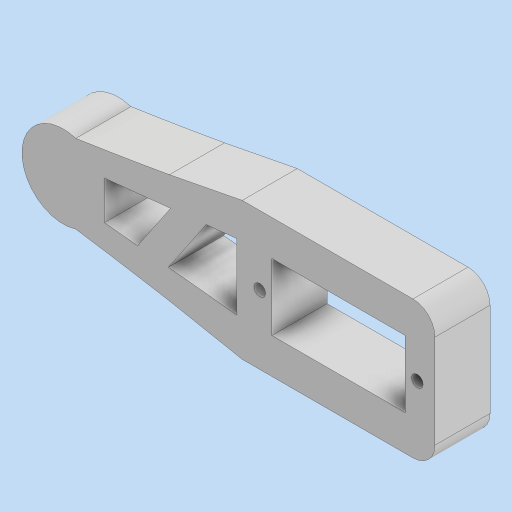
# Autodesk Inventor part: pata_inferior_v3
Saved by Autodesk Inventor 2024 (Build 280153000, 153)
## iProperties
Created: 2024-08-03
Part Number: pata_inferior_v3
Material: Generic
Document SubType Name: Modeling
Designer: MxMon
Density: 1 g/cm^3
Appearance: Default
Author: MxMon
Autodesk Inventor part; units mm, degrees
ref_plane "YZ Plane" through (0, 0, 0) normal (1, 0, 0) x (0, 1, 0)
ref_plane "XZ Plane" through (0, 0, 0) normal (0, 1, 0) x (-1, 0, 0)
ref_plane "XY Plane" through (0, 0, 0) normal (0, 0, 1) x (1, 0, 0)
sketch "Sketch1" plane through (0, 0, 0) normal (0, 0, 1) x (1, 0, 0)
  line L0 (-12.1, 6.05) -> (12.1, 6.05)
  line L1 (12.1, 6.05) -> (12.1, -6.05)
  line L2 (12.1, -6.05) -> (-12.1, -6.05)
  line L3 (-12.1, -6.05) -> (-12.1, 6.05)
  line L4 (-12.1, 6.05) -> (12.1, -6.05) construction
  line L5 (12.1, 6.05) -> (-12.1, -6.05) construction
  line L6 (-17.5, 12.5) -> (17.5, 12.5)
  line L7 (17.5, 12.5) -> (17.5, -12.5)
  line L8 (17.5, -12.5) -> (-17.5, -12.5)
  line L9 (-17.5, 12.5) -> (17.5, -12.5) construction
  line L10 (17.5, 12.5) -> (-17.5, -12.5) construction
  arc A0 (-43.9311, 7.3622) -> (-43.9311, -7.3622) centre (-42.5, 0) ccw
  line L11 (-17.5, 12.5) -> (-43.9311, 7.3622)
  line L12 (-17.5, -12.5) -> (-43.9311, -7.3622)
  point P0 (0, 0)
  point P1 (17.5, 0)
  dimension "d0" = 24.2
  dimension "d1" = 12.1
  dimension "d2" = 35
  dimension "d3" = 25
  dimension "d4" = 15
  dimension "d5" = 60
  constraints: 26 end point, 5 midpoint, 3 parallel, 2 horizontal, 2 perpendicular, 2 point on circle, 1 centre point, 1 equal length, 1 horizontal alignment, 1 tangent
  measures "d0" distance of L1.end L2.end
  measures "d1" distance of L0.end L1.end
  measures "d2" distance of L7.end L8.end
  measures "d3" distance of L6.end L7.end
  measures "d4" diameter of A0
  measures "d5" distance of A0.centre point (17.5, 0)
extrude "Extrusion1" add sketch "Sketch1" along normal blind 10
fillet "Fillet1" radius 4 2 edges at (17.5, 12.5, 5) (17.5, -12.5, 5)
sketch "Sketch2" plane through (0, 0, 10) normal (0, 0, 1) x (1, 0, 0)
  line L0 (12.1, 6.05) -> (12.1, -6.05) projected
  line L1 (-12.1, -6.05) -> (-12.1, 6.05) projected
  point P0 (0, 0)
  point P1 (14.3, 0)
  point P2 (-14.3, 0)
  dimension "d16" = 2.2
  dimension "d17" = 2.2
  constraints: 2 horizontal alignment
  measures "d16" distance from line of L0 point (14.3, 0)
  measures "d17" distance from line of point (-14.3, 0) L1
hole "Hole1" at (14.3, 0, 10) at (-14.3, 0, 10) direction (0, 0, -1) diameter 2.1 depth 8 tip angle 118
sketch "Sketch3" plane through (0, 0, 10) normal (0, 0, 1) x (1, 0, 0)
  line L0 (-18.5, 6) -> (-42.5, 3.5)
  line L1 (-18.5, -6) -> (-42.5, -3.5)
  line L2 (-42.5, -3.5) -> (-42.5, 3.5)
  line L3 (-42.5, 0) -> (-11.6221, -28.1421) construction
  line L4 (-30.5, 4.75) -> (-30.5, -4.75) construction
  arc A0 (-43.9311, 7.3622) -> (-43.9311, -7.3622) centre (-42.5, 0) ccw construction
  line L5 (-12.1, -6.05) -> (-12.1, 6.05) projected
  line L6 (-18.5, 6) -> (-18.5, -6)
  line L7 (-24.035, 5.4234) -> (-30.8838, -4.71)
  line L8 (-30.5, 4.75) -> (-36.4984, -4.1252)
  point P0 (0, 0)
  point P1 (-12.1, 0)
  point P2 (-12.1, 0)
  dimension "d27" = 7
  dimension "d31" = 24
  dimension "d32" = 6.5
  dimension "d33" = 12
  dimension "d34" = 50
  dimension "d35" = 50
  constraints: 17 end point, 5 midpoint, 3 point on line, 2 vertical, 1 coincident, 1 equal length, 1 horizontal alignment
  measures "d27" distance of L1.end L0.end
  measures "d31" horizontal distance of L1.end L1.start
  measures "d32" distance of L4.start L7.start
  measures "d33" distance of L0.start L1.start
  measures "d34" angle of L7 L0
  measures "d35" angle of L0 L8
extrude "Extrusion2" cut sketch "Sketch3" against normal blind 10
extrude "Extrusion3" add sketch "Sketch3" against normal blind 10 contours L7 L1 L8 L0
sketch "Sketch4" plane through (0, 0, 10) normal (0, 0, 1) x (1, 0, 0)
  arc A0 (-43.9311, 7.3622) -> (-43.9311, -7.3622) centre (-42.5, 0) ccw projected
  arc A1 (-47.7155, 7.1436) -> (-47.7155, -7.1436) centre (-50, 0) ccw
  line L0 (-17.5, 12.5) -> (-43.9311, 7.3622) projected
  arc A2 (-47.7155, 7.1436) -> (-30.7155, 9.9311) centre (-141.1455, 630.1772) ccw
  line L1 (-43.9311, -7.3622) -> (-17.5, -12.5) projected
  arc A3 (-30.7155, -9.9311) -> (-47.7155, -7.1436) centre (-141.1455, -630.1772) ccw
  line L2 (-18.5, 6) -> (-18.5, -6) projected
  point P0 (0, 0)
  point P1 (-18.5, 0)
  point P2 (-50, 0)
  dimension "d38" = 7.5
  dimension "d39" = 630
  dimension "d40" = 17
  constraints: 10 point on circle, 5 midpoint, 3 centre point, 2 vertical alignment, 1 equal radius, 1 horizontal alignment
  measures "d38" radius of A1
  measures "d39" radius of A2
  measures "d40" horizontal distance of point (-30.716, 9.931) A1.start
extrude "Extrusion4" add sketch "Sketch4" against normal blind 10
body "Solid1"
